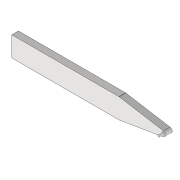
# Autodesk Inventor part: Sensor
Saved by Autodesk Inventor 2020 (Build 240168000, 168)
## iProperties
Created: 2020-04-08
Part Number: Sensor
Material: Generisch
Document SubType Name: Modeling
Designer: franz
Density: 1 g/cm^3
Appearance: Vorgabe
Author: franz
Autodesk Inventor part; units mm, degrees
ref_plane "YZ Plane" through (0, 0, 0) normal (1, 0, 0) x (0, 1, 0)
ref_plane "XZ Plane" through (0, 0, 0) normal (0, 1, 0) x (-1, 0, 0)
ref_plane "XY Plane" through (0, 0, 0) normal (0, 0, 1) x (1, 0, 0)
sketch "Skizze1" plane through (0, 0, 0) normal (0, 0, 1) x (1, 0, 0)
  line L0 (-74.0778, 7.5) -> (-74.0778, -7.5)
  line L1 (-74.0778, -7.5) -> (5.9222, -7.5)
  line L2 (6.251, -7.4728) -> (39.251, -1.9728)
  line L3 (39.251, 1.9728) -> (6.251, 7.4728)
  line L4 (5.9222, 7.5) -> (-74.0778, 7.5)
  arc A0 (6.251, 7.4728) -> (5.9222, 7.5) centre (5.9222, 5.5) ccw
  arc A1 (5.9222, -7.5) -> (6.251, -7.4728) centre (5.9222, -5.5) ccw
  arc A2 (39.251, -1.9728) -> (39.251, 1.9728) centre (38.9222, 0) ccw
  line L5 (-97.0778, 0) -> (63.9222, 0) projected
  point P0 (0, 0)
  dimension "d0" = 2
  dimension "d1" = 2
  dimension "d2" = 115
  dimension "d3" = 80
  dimension "d9" = 15
  constraints: 11 end point, 6 point on circle, 6 tangent, 3 centre point, 1 equal radius, 1 parallel, 1 perpendicular, 1 point on line, 1 symmetric about line, 1 vertical, 1 other
  measures "d0" radius of A0
  measures "d1" radius of A2
  measures "d3" distance from line of L0 A0.centre
  measures "d9" distance of L0.start L0.end
extrude "Extrusion1" add sketch "Skizze1" along normal blind 5
sketch "Skizze2" plane through (0, 0, 5) normal (0, 0, 1) x (1, 0, 0)
  arc A0 (39.251, -1.9728) -> (39.251, 1.9728) centre (38.9222, 0) ccw projected
  circle A1 centre (38.9222, 0) radius 1.25
  point P0 (0, 0)
  dimension "d6" = 2.5
  constraints: 1 centre point, 1 coincident
  measures "d6" diameter of A1
extrude "Extrusion2" add sketch "Skizze2" along normal blind 3 draft -10
